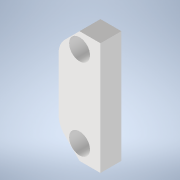
# Autodesk Inventor part: BallJointClamp
Saved by Autodesk Inventor 2020 (Build 240168000, 168)
## iProperties
Created: 2020-03-20
Part Number: BallJointClamp
Material: Generisch
Document SubType Name: Modeling
Designer: Fynn
Density: 1 g/cm^3
Appearance: Vorgabe
Author: Fynn
Autodesk Inventor part; units mm, degrees
ref_plane "YZ Plane" through (0, 0, 0) normal (1, 0, 0) x (0, 1, 0)
ref_plane "XZ Plane" through (0, 0, 0) normal (0, 1, 0) x (-1, 0, 0)
sketch "Skizze1" plane through (0, 0, 0) normal (0, 0, 1) x (1, 0, 0)
  circle A0 centre (0, 0) radius 2 projected
  circle A1 centre (0, 0) radius 1.05 projected
  circle A2 centre (0, 15.5995) radius 2 projected
  circle A3 centre (0, 15.5995) radius 1.05 projected
  line L0 (0, 18.5995) -> (4, 18.5995) projected
  line L1 (-2.8284, 15.7711) -> (0, 18.5995) projected
  arc A4 (-2.8284, 15.7711) -> (-4, 12.9427) centre (0, 12.9427) ccw projected
  line L2 (-4, 12.9427) -> (-4, 10.689) projected
  line L3 (-4, 5.0101) -> (-4, 2.7564) projected
  arc A5 (-4, 2.7564) -> (-2.8284, -0.072) centre (0, 2.7564) ccw projected
  line L4 (0, -2.9005) -> (-2.8284, -0.072) projected
  line L5 (4, -2.9005) -> (0, -2.9005) projected
  line L6 (4, 18.5995) -> (4, -2.9005) projected
  line L7 (-4, 10.689) -> (-4, 5.0101)
  point P0 (0, 0)
  constraints: 2 end point, 1 vertical
extrude "Extrusion1" add sketch "Skizze1" along normal blind 4 contours L0 L6 L5 L4 A5 L3 L7 L2 A4 L1
sketch "Skizze2" plane through (0, 0, 4) normal (0, 0, 1) x (1, 0, 0)
  line L0 (0, 18.5995) -> (-2.8284, 15.7711) projected
  arc A0 (-2.8284, 15.7711) -> (-4, 12.9427) centre (0, 12.9427) ccw projected
  line L1 (-4, 12.9427) -> (-4, 2.7564) projected
  arc A1 (-4, 2.7564) -> (-2.8284, -0.072) centre (0, 2.7564) ccw projected
  line L2 (-2.8284, -0.072) -> (0, -2.9005) projected
  line L3 (0, -2.9005) -> (4, -2.9005) projected
  line L4 (4, -2.9005) -> (4, 18.5995) projected
  line L5 (4, 18.5995) -> (0, 18.5995) projected
  circle A2 centre (0, 15.5995) radius 2 projected
  circle A3 centre (0, 0) radius 2 projected
  circle A4 centre (0, 15.5995) radius 1.05
  circle A5 centre (0, 0) radius 1.05
  point P0 (0, 0)
  dimension "d2" = 2.1
  dimension "d3" = 2.1
  constraints: 2 centre point, 2 coincident
  measures "d2" diameter of A4
  measures "d3" diameter of A5
extrude "Extrusion2" add sketch "Skizze2" along normal blind 2 contours L5 L4 L3 L2 A1 L1 A0 L0 | A2 | A3
sketch "Skizze3" plane through (0, 0, 0) normal (0, 0, -1) x (-1, 0, 0)
  line L0 (0, -2.9005) -> (-4, -2.9005) projected
  line L1 (-4, -2.9005) -> (-4, 7.8495)
  line L2 (-4, -2.9005) -> (-4, 18.5995) projected
  line L3 (-4, 7.8495) -> (1, 7.8495)
  circle A0 centre (1, 7.8495) radius 4.25
  line L4 (1, 7.8495) -> (5.25, 7.8495)
  line L5 (4, 12.9427) -> (4, 2.7564) projected
  point P0 (0, 0)
  point P1 (4, 7.8495)
  point P2 (4, 10.8599)
  point P3 (-3.25, 7.8495)
  dimension "d7" = 8.5
  dimension "d8" = 3
  constraints: 6 end point, 2 horizontal, 1 coincident, 1 midpoint, 3 other
  measures "d8" distance from line of L5 L3.end
revolve "Umdrehung1" cut sketch "Skizze3" angle 360 about axis through (4, 7.8495, 0) along (-1, 0, 0) picked at (3, 8.853) contours A0 L5 L4 L3
sketch "Skizze4" plane through (0, 0, 0) normal (0, 0, -1) x (-1, 0, 0)
  line L0 (-4.7683, -3.7941) -> (5.6191, -3.7941)
  line L1 (5.6191, -3.7941) -> (5.6191, 20.4958)
  line L2 (5.6191, 20.4958) -> (-4.7683, 20.4958)
  line L3 (-4.7683, 20.4958) -> (-4.7683, -3.7941)
  point P0 (0, 0)
  constraints: 8 end point, 2 parallel, 1 horizontal, 1 perpendicular
extrude "Extrusion3" cut sketch "Skizze4" against normal blind 1
sketch "Skizze5" plane through (4, -2.9005, 6) normal (1, 0, 0) x (0, 0, -1)
  line L0 (5, 0) -> (5, 21.5) projected
  line L1 (5, 21.5) -> (0, 21.5) projected
  line L2 (0, 0) -> (0, 21.5) projected
  line L3 (5, 0) -> (0, 0) projected
  point P0 (6, 2.9005)
extrude "Extrusion4" cut sketch "Skizze5" against normal blind 1
sketch "Skizze6" plane through (0, 0, 1) normal (0, 0, -1) x (-1, 0, 0)
  line L0 (2.8284, -0.072) -> (0, -2.9005) projected
  line L1 (0, -2.9005) -> (0.4894, -2.9005)
  arc A0 (2.8284, -0.072) -> (4, 2.7564) centre (0, 2.7564) ccw projected
  line L2 (0.4894, -2.9005) -> (4, -2.9005)
  line L3 (4, -2.9005) -> (4, 2.7564)
  point P0 (0, 0)
  point P1 (3.7092, 1.2591)
  constraints: 6 end point, 2 horizontal, 1 perpendicular, 1 point on circle
extrude "Extrusion5" add sketch "Skizze6" against normal up to surface (5 mm away)
ref_plane "Arbeitsebene1" through (0, 7.8495, 6) normal (0, 1, 0) x (1, 0, 0)
sketch "Skizze9" plane through (0, 0, 1) normal (0, 0, -1) x (-1, 0, 0)
  circle A0 centre (0, 0) radius 2.5
  dimension "d24" = 5
  constraints: 1 centre point, 1 coincident
  measures "d24" diameter of A0
extrude "Extrusion8" cut sketch "Skizze9" against normal up to surface (3 mm away)
sketch "Skizze10" plane through (0, 0, 1) normal (0, 0, -1) x (-1, 0, 0)
  line L0 (0.6938, -3.6003) -> (3.1846, -0.5858)
  line L1 (3.1846, -0.5858) -> (4, 4.2826)
  line L2 (4, -2.9005) -> (4, 5.0101) projected
  line L3 (4, -2.9005) -> (-3, -2.9005) projected
  point P0 (0, 0)
  point P1 (1.272, -2.9005)
  constraints: 4 end point, 1 point on line
extrude "Extrusion9" cut sketch "Skizze10" against normal through all
mirror "Spiegeln3" about plane through (0, 7.8495, 6) normal (0, 1, 0) of "Extrusion5", "Extrusion8", "Extrusion9"
sketch "Skizze11" plane through (3, 18.5995, 6) normal (0, 1, 0) x (1, 0, 0)
  line L0 (-7, 2.9896) -> (-7, 5) projected
  line L1 (-7.4841, 2.5704) -> (-4.5207, -0.7469)
  line L2 (-4.5207, -0.7469) -> (-5.1252, -3.6367)
  line L3 (-5.1252, -3.6367) -> (-9.8579, -0.57)
  line L4 (-9.8579, -0.57) -> (-7.4841, 2.5704)
  point P0 (-3, 6)
  constraints: 8 end point, 1 point on line
extrude "Extrusion10" cut sketch "Skizze11" against normal through all
chamfer "Fase2" distance 0.5 angle 45 1 edges at (-2.188, 7.8495, 6)
